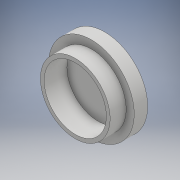
# Autodesk Inventor part: CapForPh
Saved by Autodesk Inventor 2018.1 (Build 221171000, 171)
## iProperties
Created: 2017-07-24
Part Number: CapForPh
Material: Generic
Document SubType Name: Modeling
Designer: steele
Density: 1 g/cm^3
Appearance: Default
Author: steele
Autodesk Inventor part; units mm, degrees
ref_plane "YZ Plane" through (0, 0, 0) normal (1, 0, 0) x (0, 1, 0)
ref_plane "XZ Plane" through (0, 0, 0) normal (0, 1, 0) x (-1, 0, 0)
ref_plane "XY Plane" through (0, 0, 0) normal (0, 0, 1) x (1, 0, 0)
sketch "Sketch2" plane through (0, 0, 0) normal (0, 0, 1) x (1, 0, 0)
  line L0 (0, 0) -> (0, 11) construction
  line L1 (0, 11) -> (-16, 11)
  line L2 (-16, 11) -> (-16, 6)
  line L3 (-16, 6) -> (-13, 6)
  line L4 (-13, 6) -> (-13, 0)
  line L5 (-13, 0) -> (-11.6, 0)
  line L6 (0, 0) -> (-13, 0) construction
  line L7 (-11.6, 0) -> (-11.6, 6)
  line L8 (0, 11) -> (0, 8.5)
  line L9 (-11.6, 8.5) -> (-11.6, 6)
  line L10 (-11.6, 8.5) -> (0, 8.5)
  dimension "d4" = 16
  dimension "d5" = 5
  dimension "d6" = 6
  dimension "d8" = 13
  dimension "d11" = 1.4
  constraints: 22 end point, 5 perpendicular, 3 vertical, 2 point on line, 1 collinear, 1 horizontal, 1 parallel
  measures "d4" distance of L0.end L1.end
  measures "d5" distance of L1.end L2.end
  measures "d6" distance of L3.end L4.end
  measures "d8" distance between parallel lines of L0 L4
  measures "d11" distance between parallel lines of L7 L4
revolve "Revolution1" add sketch "Sketch2" angle 360 about axis through (0, 0, 0) along (0, 1, 0)
body "Solid1"
